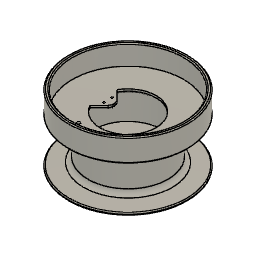
Windlass Drum v1 (Autodesk Fusion 360 design; units mm, degrees)
Autodesk Fusion 360 part; units mm, degrees
sketch "Sketch1" plane through (0, 0, 0) normal (0, 1, 0) x (1, 0, 0) in component "Windlass drum"
  circle A0 centre (0, 0) radius 75.565
  circle A1 centre (0, 0) radius 6.35
  circle A2 centre (0, 0) radius 31.369
  dimension "d1" = 151.13
  dimension "d2" = 12.7
  dimension "d3" = 62.738
  constraint coincident A0.centre A1.centre
  measures "d1" diameter of A0
  measures "d2" diameter of A1
  measures "d3" diameter of A2
extrude "Extrude1" add sketch "Sketch1" along normal blind 86.8172 contours A0 | A1 | A2 makes body 1 in component "Windlass drum"
extrude "Extrude2" cut sketch "Sketch1" along normal blind 9.525 contours A2 bodies 1 in component "Windlass drum"
extrude "Extrude3" cut sketch "Sketch1" along normal through all contours A1 bodies 1 in component "Windlass drum"
sketch "Sketch2" plane through (0, 86.8172, 0) normal (0, 1, 0) x (-1, 0, 0) in component "Windlass drum"
  circle A0 centre (0, 0) radius 6.35
  circle A1 centre (0, 0) radius 75.565
  circle A2 centre (0, 0) radius 70.8025
  circle A3 centre (0, 0) radius 42.8625
  circle A4 centre (0, 0) radius 47.625
  dimension "d9" = 141.605
  dimension "d10" = 85.725
  dimension "d11" = 95.25
  constraint concentric A0 A2
  constraint concentric A2 A3
  constraint concentric A2 A4
  measures "d9" diameter of A2
  measures "d10" diameter of A3
  measures "d11" diameter of A4
extrude "Extrude4" cut sketch "Sketch2" against normal blind 25.4 contours A0 | A2 | A3 | A4 bodies 1 in component "Windlass drum"
extrude "Extrude5" cut sketch "Sketch2" against normal blind 66.3702 contours A0 | A3 bodies 1 in component "Windlass drum"
sketch "Sketch3" plane through (0, 0, 0) normal (1, 0, 0) x (0, 0, -1) in component "Windlass drum"
  line L0 (75.565, 0) -> (-75.565, 0)
  line L1 (70.8025, 86.8172) -> (-70.8025, 86.8172)
  line L2 (75.565, 86.8172) -> (-75.565, 86.8172)
  line L3 (0, 86.8172) -> (0, 0) construction
  line L4 (50.8, 86.8172) -> (50.8, 0) construction
  line L5 (-50.8, 86.8172) -> (-50.8, 0) construction
  line L6 (75.565, 57.6072) -> (50.8, 53.7972)
  line L7 (75.565, 3.048) -> (50.8, 6.858)
  line L8 (50.8, 53.7972) -> (50.8, 6.858)
  line L9 (75.565, 57.6072) -> (75.565, 86.8172)
  line L10 (75.565, 3.048) -> (75.565, 0)
  line L11 (75.565, 57.6072) -> (75.565, 3.048)
  point P0 (0, 86.8172)
  point P1 (75.565, 3.048)
  point P2 (75.565, 57.6072)
  point P3 (50.8, 6.858)
  dimension "d18" = 50.8
  dimension "d19" = 50.8
  dimension "d20" = 3.048
  dimension "d21" = 29.21
  dimension "d23" = 3.81
  dimension "d24" = 3.81
  constraint coincident P0 L3.start
  constraint coincident L3.end origin
  constraint coincident L1 L4.start
  constraint coincident L0 L4.end
  constraint perpendicular L0 L4
  constraint coincident L2 L5.start
  constraint coincident L0 L5.end
  constraint perpendicular L0 L5
  constraint vertical P1 P2
  constraint coincident L4 P3
  constraint coincident P2 L6.start
  constraint coincident L4 L6.end
  constraint coincident P1 L7.start
  constraint coincident P3 L7.end
  constraint parallel L4 L8
  constraint coincident L2.start L9.end
  constraint perpendicular L2 L9
  constraint coincident L0.start L10.end
  measures "d18" distance of L3 L4
  measures "d19" distance of L3 L5
  measures "d20" distance of L0 P1
  measures "d21" distance of L2.start P2
  measures "d23" vertical distance of P2 L6.end
  measures "d24" vertical distance of P1 P3
revolve "Revolve1" cut sketch "Sketch3" angle 360 about axis through (0, 0, 0) along (0, -1, 0) bodies 1 in component "Windlass drum"
sketch "Sketch4" plane through (0, 61.4172, 0) normal (0, 1, 0) x (-1, 0, 0) in component "Windlass drum"
  circle A0 centre (0, 0) radius 70.8025
  circle A1 centre (25.4, 0) radius 3.3734
  circle A2 centre (0, 0) radius 6.35
  circle A3 centre (0, 0) radius 42.8625
  circle A4 centre (0, 0) radius 47.625
  line L0 (0, 0, 25.4) -> (0, 0, -61.4172)
  circle A5 centre (19.05, 43.649) radius 2.0193
  line L1 (0, 70.8025) -> (0, -70.8025) construction
  circle A6 centre (-19.05, 43.649) radius 2.0193
  circle A7 centre (0, 61.9125) radius 6.35
  circle A8 centre (0, 0) radius 35.56
  line L2 (17.78, 1.1797) -> (17.78, -30.7959)
  circle A9 centre (25.4, 5.08) radius 1.27
  circle A10 centre (25.4, -5.08) radius 1.27
  line L3 (25.4, 9.1096) -> (25.4, -10.3282) construction
  line L4 (19.6399, 5.6699) -> (31.1401, 17.1701)
  line L5 (17.78, 3.81) -> (35.6219, 3.81) construction
  arc A11 (19.6399, 5.6699) -> (17.78, 1.1797) centre (24.13, 1.1797) ccw
  line L6 (-2.5, 0) -> (-20, 0)
  line L7 (19.6399, -5.6699) -> (31.1401, -17.1701)
  arc A12 (17.78, -1.1797) -> (19.6399, -5.6699) centre (24.13, -1.1797) ccw
  line L8 (17.78, -1.1797) -> (17.78, 30.7959)
  dimension "d26" = 6.7469
  dimension "d27" = 25.4
  dimension "d28" = 4.0386
  dimension "d29" = 19.05
  dimension "d30" = 12.7
  dimension "d31" = 8.89
  dimension "d57" = 25.4
  dimension "d58" = 95.25
  dimension "d59" = 71.12
  dimension "d60" = 17.78
  dimension "d61" = 2.54
  dimension "d62" = 2.54
  dimension "d64" = 5.08
  dimension "d65" = 45
  dimension "d66" = 6.35
  dimension "d73" = 5.08
  constraint coincident A4 A5.centre
  constraint coincident A0 L1.start
  constraint coincident A0 L1.end
  constraint vertical L1
  constraint symmetric A5 L1 A6
  constraint coincident L1 A7.centre
  constraint concentric A4 A8
  constraint coincident A8 L2.end
  constraint parallel L1 L2
  constraint vertical L3
  constraint coincident A9.centre L3
  constraint coincident A10.centre L3
  constraint horizontal L5
  constraint coincident L2 L5.start
  constraint coincident A8 L4.end
  constraint coincident L5.start L4
  constraint tangent L4 A11
  constraint tangent L2 A11
  constraint symmetric L2.end L6 L8.end
  constraint symmetric L4.end L6 L7.end
  constraint symmetric L4.start L6 L7.start
  constraint symmetric L2.start L6 A12.start
  constraint symmetric A11 L6 A12
  measures "d26" diameter of A1
  measures "d28" diameter of A5
  measures "d29" distance of A5.centre L1
  measures "d30" diameter of A7
  measures "d31" distance of L1.start A7.centre
  measures "d57" distance of A0.centre A1.centre
  measures "d58" diameter of A4
  measures "d59" diameter of A8
  measures "d60" distance of A0.centre L2
  measures "d61" diameter of A9
  measures "d62" diameter of A10
  measures "d64" distance of A1.centre A10.centre
  measures "d65" angle of L4 L5
  measures "d66" radius of A11
  measures "d73" vertical distance of A9.centre A0.centre
extrude "Extrude7" cut sketch "Sketch4" against normal blind 10.922 contours A7 bodies 1 in component "Windlass drum"
extrude "Extrude8" cut sketch "Sketch4" against normal blind 64.77 contours A1 bodies 1 in component "Windlass drum"
extrude "Extrude9" cut sketch "Sketch4" against normal blind 25.4 contours A4 A5 | A4 A5 | A4 A6 | A4 A6 bodies 1 in component "Windlass drum"
fillet "Fillet1" radius 6.35 2 edges at (-47.3622, 6.858, -18.3701) (-47.3622, 53.7972, -18.3701) on bodies 1 in component "Windlass drum"
fillet "Fillet2" radius 1.27 2 edges at (-70.4513, 86.8172, 27.3255) (66.0111, 86.8172, 25.6033) on bodies 1 in component "Windlass drum"
fillet "Fillet3" radius 1.27 3 edges at (-70.4513, 57.6072, 27.3255) (-70.4513, 3.048, -27.3255) (-70.4513, 0, 27.3255) on bodies 1 in component "Windlass drum"
fillet "Fillet4" radius 2.54 4 edges at (5.9203, 61.4172, 64.2088) (0.0137, 54.4978, 55.5625) (-3.1809, 56.3637, 67.4071) (5.1414, 54.9687, 58.1882) on bodies 1 in component "Windlass drum"
ref_plane "WorkPlane1" through (0, 20.447, 0) normal (0, 1, 0) x (0, 0, 1)
ref_plane "WorkPlane2" through (0, 61.4172, 0) normal (0, 1, 0) x (0, 0, 1)
split "Split1" by plane through (0, 20.447, 0) normal (0, 1, 0) bodies 1 makes body 2 at (0, 76.5971, -75.565) in component "Windlass drum"
split "Split2" by plane through (0, 61.4172, 0) normal (0, 1, 0) bodies 2 makes body 3 at (75.1895, 69.4605, -7.5238) in component "Windlass drum"
sketch "Sketch1 (2)" plane through (0, 0, 0) normal (1, 0, 0) x (0, 0, -1)
  line L0 (-50.8, 12.3058) -> (50.8, 12.3058)
  line L1 (50.8, 20.447) -> (-50.8, 20.447)
  line L2 (-50.8, 20.447) -> (-46.482, 20.447)
  line L3 (-46.482, 20.447) -> (-46.482, 12.3058)
  line L4 (-46.482, 12.3058) -> (-50.8, 12.3058)
  line L5 (-50.8, 12.3058) -> (-50.8, 20.447)
  line L6 (-46.5101, 20.447) -> (-46.6709, 12.3058)
  line L7 (75.565, 61.4172) -> (-75.565, 61.4172)
  line L8 (75.565, 85.5472) -> (-75.565, 85.5472)
  line L9 (-75.565, 61.4172) -> (-73.025, 61.4172)
  line L10 (-73.025, 61.4172) -> (-73.025, 58.6988)
  line L11 (-73.025, 58.6988) -> (-75.565, 58.6988)
  line L12 (-75.565, 58.6988) -> (-75.565, 61.4172)
  line L13 (-73.0322, 61.4172) -> (-73.0909, 58.6988)
  dimension "d50" = 4.318
  dimension "d53" = 2.54
  dimension "d54" = 2.7184
  constraint horizontal L2
  constraint vertical L3
  constraint horizontal L4
  constraint vertical L5
  constraint coincident L1.end L2.start
  constraint coincident L1 L6.start
  constraint coincident L0 L6.end
  constraint coincident L4 L6.end
  constraint horizontal L9
  constraint vertical L10
  constraint horizontal L11
  constraint vertical L12
  constraint coincident L7.end L9.start
  constraint coincident L7 L13.start
  constraint coincident L11 L13.end
  measures "d50" distance of L1.end L2.end
  measures "d53" distance of L7.end L9.end
  measures "d54" distance of L7.end L11.end
revolve "Revolve2" cut sketch "Sketch1 (2)" angle 360 about axis through (0, 1.75, 0) along (0, 1, 0) contours L0 L1 L2 L4 L5 L6 | L0 L1 L2 L3 L4 L6 bodies 1 in component "Windlass drum"
revolve "Revolve3" add sketch "Sketch1 (2)" angle 360 about axis through (0, 1.75, 0) along (0, 1, 0) contours L0 L1 L2 L4 L5 L6 bodies 2 in component "Windlass drum"
revolve "Revolve4" cut sketch "Sketch1 (2)" angle 360 about axis through (0, 1.75, 0) along (0, 1, 0) contours L7 L9 L10 L11 L13 | L7 L9 L11 L12 L13 bodies 2 in component "Windlass drum"
revolve "Revolve5" add sketch "Sketch1 (2)" angle 360 about axis through (0, 1.75, 0) along (0, 1, 0) contours L7 L9 L11 L12 L13 bodies 3 in component "Windlass drum"
extrude "Extrude10" add sketch "Sketch4" against normal blind 5.08 contours A1 | A3 | A8 L2 L4 A11 L7 A12 L8 bodies 2 in component "Windlass drum"
fillet "Fillet6" radius 2.54 6 edges at (35.56, 56.3372, 0) (-25.39, 56.3372, -11.42) (-18.2634, 56.3372, -3.6098) (-17.78, 56.3372, 0) (-18.2634, 56.3372, 3.6098) (-25.39, 56.3372, 11.42) on bodies 2 in component "Windlass drum"
component "Windlass drum" placed x (1, 0, 0) y (0, 1, 0) z (0, 0, 1) at (0, 0, 0)
equation "d19 = d18"
equation "d26 = ( 17 / 64 ) * 1 in"
equation "d64 = d73"
named bodies: "Windlass drum inner", "Windlass drum outer", "Windlass drum rim"
